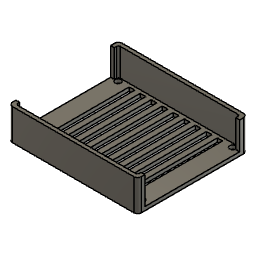
back_side (Autodesk Fusion 360 design; units mm, degrees)
Autodesk Fusion 360 part; units mm, degrees
sketch "Sketch1" plane through (0, 0, 0) normal (0, 1, 0) x (1, 0, 0)
other "Base Mesh Feature1"
sketch "Sketch2" plane through (0, 0, 0) normal (1, 0, 0) x (0, 0, -1)
other "Body->Comp1"
sketch "Sketch3" plane through (0, 20, 0) normal (0, 1, 0) x (1, 0, 0)
  line L0 (-70.2, 57.4) -> (70.2, 57.4)
  line L1 (70.2, 57.4) -> (70.2, -62)
  line L2 (70.2, -62) -> (-70.2, -62)
  line L3 (-70.2, -62) -> (-70.2, 57.4)
  circle A0 centre (-62.365, -49.3376) radius 3.25
  circle A1 centre (62.2857, -49.3492) radius 3.25
  circle A2 centre (-62.4, 49.35) radius 3.25
  circle A3 centre (62.2, 49.4) radius 3.25
  dimension "d1" = 6.5
  dimension "d2" = 6.5
  dimension "d3" = 6.5
  dimension "d4" = 6.5
  constraint horizontal L0
  constraint vertical L1
  constraint horizontal L2
  constraint vertical L3
  measures "d1" diameter of A0
  measures "d2" diameter of A1
  measures "d3" diameter of A2
  measures "d4" diameter of A3
extrude "Extrude1" add sketch "Sketch3" along normal blind 4
fillet "Fillet1" radius 4 1 edges at (-70.2, 22, -57.4)
fillet "Fillet2" radius 4 1 edges at (70.2, 22, -57.4)
fillet "Fillet3" radius 4 1 edges at (70.2, 22, 62)
fillet "Fillet4" radius 4 1 edges at (-70.2, 22, 62)
sketch "Sketch4" plane through (0, 24, 0) normal (0, 1, 0) x (-1, 0, 0)
  arc A0 (70.2, 58) -> (66.2, 62) centre (66.2, 58) ccw
  line L0 (66.2, 62) -> (-66.2, 62)
  arc A1 (-66.2, 62) -> (-70.2, 58) centre (-66.2, 58) ccw
  line L1 (-70.2, 58) -> (-70.2, -53.4)
  arc A2 (-70.2, -53.4) -> (-66.2, -57.4) centre (-66.2, -53.4) ccw
  line L2 (-66.2, -57.4) -> (66.2, -57.4)
  arc A3 (66.2, -57.4) -> (70.2, -53.4) centre (66.2, -53.4) ccw
  line L3 (70.2, -53.4) -> (70.2, 58)
  circle A4 centre (62.365, 49.3376) radius 3.25
  circle A5 centre (-62.2, -49.4) radius 3.25
  circle A6 centre (-62.2857, 49.3492) radius 3.25
  circle A7 centre (62.4, -49.35) radius 3.25
  line L4 (-64.0005, 58) -> (64.2, 58)
  line L5 (66.2, 56) -> (66.2, -51.4)
  line L6 (64.2, -53.4) -> (-64.0005, -53.4)
  line L7 (-66.0005, -51.4) -> (-66.0005, 56)
  arc A8 (64.2, -53.4) -> (66.2, -51.4) centre (64.2, -51.4) ccw
  arc A9 (-66.0005, -51.4) -> (-64.0005, -53.4) centre (-64.0005, -51.4) ccw
  arc A10 (-64.0005, 58) -> (-66.0005, 56) centre (-64.0005, 56) ccw
  arc A11 (66.2, 56) -> (64.2, 58) centre (64.2, 56) ccw
  dimension "d15" = 2
  dimension "d16" = 2
  dimension "d17" = 2
  dimension "d18" = 2
  constraint horizontal L4
  constraint vertical L5
  constraint horizontal L6
  constraint vertical L7
  constraint tangent L5 A8
  constraint tangent L6 A8
  constraint tangent L6 A9
  constraint tangent L7 A9
  constraint tangent L4 A10
  constraint tangent L7 A10
  constraint tangent L4 A11
  constraint tangent L5 A11
  measures "d15" radius of A8
  measures "d16" radius of A9
  measures "d17" radius of A10
  measures "d18" radius of A11
extrude "Extrude2" add sketch "Sketch4" along normal blind 30 contours A0 L0 A1 L1 A2 L2 A3 L3
sketch "Sketch5" plane through (0, 0, 0) normal (0, 1, 0) x (1, 0, 0)
  line L0 (3, 50) -> (-3, 50)
  line L1 (-3, 50) -> (-3, -50)
  line L2 (-3, -50) -> (3, -50)
  line L3 (3, -50) -> (3, 50)
  line L4 (-9, 50) -> (-15, 50)
  line L5 (-15, 50) -> (-15, -50)
  line L6 (-15, -50) -> (-9, -50)
  line L7 (-9, -50) -> (-9, 50)
  line L8 (-21, 50) -> (-27, 50)
  line L9 (-27, 50) -> (-27, -50)
  line L10 (-27, -50) -> (-21, -50)
  line L11 (-21, -50) -> (-21, 50)
  line L12 (-33, 50) -> (-39, 50)
  line L13 (-39, 50) -> (-39, -50)
  line L14 (-39, -50) -> (-33, -50)
  line L15 (-33, -50) -> (-33, 50)
  line L16 (-45, 50) -> (-51, 50)
  line L17 (-51, 50) -> (-51, -50)
  line L18 (-51, -50) -> (-45, -50)
  line L19 (-45, -50) -> (-45, 50)
  line L20 (9, 50) -> (15, 50)
  line L21 (15, 50) -> (15, -50)
  line L22 (15, -50) -> (9, -50)
  line L23 (9, -50) -> (9, 50)
  line L24 (21, 50) -> (27, 50)
  line L25 (27, 50) -> (27, -50)
  line L26 (27, -50) -> (21, -50)
  line L27 (21, -50) -> (21, 50)
  line L28 (33, 50) -> (39, 50)
  line L29 (39, 50) -> (39, -50)
  line L30 (39, -50) -> (33, -50)
  line L31 (33, -50) -> (33, 50)
  line L32 (45, 50) -> (50.6614, 50)
  line L33 (50.6614, 50) -> (50.6614, -50)
  line L34 (50.6614, -50) -> (45, -50)
  line L35 (45, -50) -> (45, 50)
  dimension "d21" = 6
  dimension "d22" = 100
  dimension "d23" = 6
  dimension "d24" = 100
  dimension "d25" = 6
  dimension "d26" = 100
  dimension "d27" = 6
  dimension "d28" = 100
  dimension "d29" = 6
  dimension "d30" = 100
  dimension "d31" = 6
  dimension "d32" = 100
  dimension "d33" = 6
  dimension "d34" = 100
  dimension "d35" = 100
  constraint horizontal L0
  constraint vertical L1
  constraint horizontal L2
  constraint vertical L3
  constraint horizontal L4
  constraint vertical L5
  constraint horizontal L6
  constraint vertical L7
  constraint horizontal L8
  constraint vertical L9
  constraint horizontal L10
  constraint vertical L11
  constraint horizontal L12
  constraint vertical L13
  constraint horizontal L14
  constraint vertical L15
  constraint horizontal L16
  constraint vertical L17
  constraint horizontal L18
  constraint vertical L19
  constraint horizontal L20
  constraint vertical L21
  constraint horizontal L22
  constraint vertical L23
  constraint horizontal L24
  constraint vertical L25
  constraint horizontal L26
  constraint vertical L27
  constraint horizontal L28
  constraint vertical L29
  constraint horizontal L30
  constraint vertical L31
  constraint horizontal L32
  constraint vertical L33
  constraint horizontal L34
  constraint vertical L35
  measures "d21" distance of L4.start L4.end
  measures "d22" distance of L4.start L6.end
  measures "d23" distance of L8.start L8.end
  measures "d24" distance of L8.start L10.end
  measures "d25" distance of L12.start L12.end
  measures "d26" distance of L12.start L14.end
  measures "d27" distance of L16.start L16.end
  measures "d28" distance of L16.start L18.end
  measures "d29" distance of L20.start L20.end
  measures "d30" distance of L20.start L22.end
  measures "d31" distance of L24.start L24.end
  measures "d32" distance of L24.start L26.end
  measures "d33" distance of L28.start L28.end
  measures "d34" distance of L28.start L30.end
  measures "d35" distance of L32.start L34.end
extrude "Extrude3" cut sketch "Sketch5" along normal blind 84 contours L4 L5 L6 L7 | L8 L9 L10 L11 | L12 L13 L14 L15 | L16 L17 L18 L19 | L20 L21 L22 L23 | L24 L25 L26 L27 | L28 L29 L30 L31 | L32 L33 L34 L35
sketch "Sketch6" plane through (0, 0, 0) normal (0, 1, 0) x (1, 0, 0)
  line L0 (-3, 50) -> (3, 50)
  line L1 (3, 50) -> (3, -50)
  line L2 (3, -50) -> (-3, -50)
  line L3 (-3, -50) -> (-3, 50)
  dimension "d38" = 100
  constraint horizontal L0
  constraint vertical L1
  constraint horizontal L2
  constraint vertical L3
  measures "d38" distance of L0.start L2.end
extrude "Extrude4" cut sketch "Sketch6" along normal blind 202
ref_plane "WorkPlane1" through (70.2, 37, 2.3) normal (1, 0, 0) x (0, 0, -1)
sketch "Sketch7" plane through (70.2, 0, 0) normal (1, 0, 0) x (0, 0, -1)
  line L0 (-54, 24) -> (49, 24)
  line L1 (49, 24) -> (49, 55)
  line L2 (49, 55) -> (-54, 55)
  line L3 (-54, 55) -> (-54, 24)
  constraint horizontal L0
  constraint vertical L1
  constraint horizontal L2
  constraint vertical L3
extrude "Extrude5" cut sketch "Sketch7" against normal blind 179
component "Inkplate6Color_V1" placed x (1, 0, 0) y (0, 1, 0) z (0, 0, 1) at (0, 0, 0)
